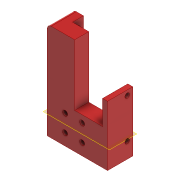
# Autodesk Inventor part: Collector mount adapter
Saved by Autodesk Inventor 2020 (Build 240168000, 168)
## iProperties
Created: 2020-01-01
Part Number: Collector mount adapter
Material: Generic
Document SubType Name: Modeling
Designer: ball
Density: 1 g/cm^3
Appearance: Default
Author: ball
Autodesk Inventor part; units mm, degrees
ref_plane "YZ Plane" through (0, 0, 0) normal (1, 0, 0) x (0, 1, 0)
ref_plane "XZ Plane" through (0, 0, 0) normal (0, 1, 0) x (-1, 0, 0)
ref_plane "Work Plane1" through (0, 0, 0) normal (0, 0, 1) x (1, 0, 0)
sketch "Sketch1" plane through (0, 0, 0) normal (0, 0, 1) x (1, 0, 0)
  line L0 (-13.625, 22.3146) -> (-10.375, 22.3146) construction
  line L1 (3.2502, 80.8) -> (3.2502, 93.5) construction
  line L2 (14.75, 68.1) -> (10.0002, 68.1) construction
  circle A0 centre (12.375, 55.8) radius 3.5 construction
  circle A1 centre (12.375, 47.8) radius 1.7 construction
  line L3 (-18.004, 18.76) -> (18.004, 18.76)
  line L4 (18.004, 18.76) -> (18.004, 47.8)
  line L5 (18.004, 47.8) -> (-4.75, 47.8)
  line L6 (-18.004, 47.8) -> (-18.004, 18.76)
  line L7 (-1.55, 84.1622) -> (-1.55, 90.1378) construction
  line L8 (-4.75, 85.6895) -> (-4.75, 88.6105) construction
  line L9 (17.75, 97.5) -> (-17.75, 97.5) construction
  line L10 (-4.75, 47.8) -> (-4.75, 97.5)
  line L11 (-4.75, 97.5) -> (-18.004, 97.5)
  line L12 (-18.004, 97.5) -> (-18.004, 47.8)
  point P0 (0, 0)
  dimension "d51" = 18.004
  dimension "d52" = 18.004
  dimension "d78" = 97.5
  dimension "d79" = 78.74
  constraints: 26 end point, 4 horizontal, 3 parallel, 3 vertical, 2 centre point, 1 perpendicular, 1 point on line, 16 other
  measures "d51" distance from line of L6 point (0, 0)
  measures "d52" distance from line of L4 point (0, 0)
  measures "d78" distance from line of L9 point (0, 0)
  measures "d79" distance between parallel lines of L3 L9
extrude "Base shape" add sketch "Sketch1" along normal blind 11.4808
sketch "Sketch4" plane through (-18.004, 18.76, 0) normal (-1, 0, 0) x (0, 0, 1)
  line L0 (0, 78.74) -> (11.4808, 78.74) projected
  line L1 (11.4808, 78.74) -> (-8.9916, 78.74)
  line L2 (-8.9916, 78.74) -> (-8.9916, 0)
  line L3 (-8.9916, 0) -> (11.4808, 0)
  line L4 (11.4808, 0) -> (11.4808, 78.74)
  circle A0 centre (-4.4958, 72.0852) radius 1.9
  line L5 (0, 78.74) -> (0, 0) projected
  circle A1 centre (-4.4958, 44.8056) radius 1.9
  circle A2 centre (-4.4958, 12.74) radius 1.9
  point P0 (0, -18.76)
  dimension "d29" = 3.8
  dimension "d30" = 6.6548
  dimension "d32" = 4.4958
  dimension "d33" = 3.8
  dimension "d34" = 3.8
  dimension "d35" = 33.9344
  dimension "d36" = 66
  dimension "d53" = 8.9916
  dimension "d54" = 4.4958
  dimension "d55" = 4.4958
  constraints: 8 end point, 3 centre point, 2 parallel, 1 horizontal, 1 perpendicular
  measures "d29" diameter of A0
  measures "d30" distance from line of L1 A0.centre
  measures "d32" distance from line of L2 A0.centre
  measures "d33" diameter of A1
  measures "d34" diameter of A2
  measures "d35" distance from line of L1 A1.centre
  measures "d36" distance from line of L1 A2.centre
  measures "d53" distance between parallel lines of L2 L5
  measures "d54" distance from line of L2 A1.centre
  measures "d55" distance from line of L2 A2.centre
extrude "Non Pulley Side" add sketch "Sketch4" along normal blind 9
sketch "Sketch5" plane through (18.004, 18.76, 0) normal (1, 0, 0) x (0, 0, -1)
  line L0 (0, 0) -> (-11.4808, 0) projected
  line L1 (0, 78.74) -> (8.9916, 78.74) projected
  line L2 (-11.4808, 0) -> (8.9916, 0)
  line L3 (8.9916, 0) -> (8.9916, 48.815)
  line L4 (8.9916, 78.74) -> (-9.652, 78.74) construction
  line L5 (-11.4808, 48.815) -> (-11.4808, 0)
  circle A0 centre (4.4958, 12.74) radius 1.9
  circle A1 centre (4.4958, 44.815) radius 1.9
  line L6 (8.9916, 78.74) -> (8.9916, 0) projected
  line L7 (8.9916, 48.815) -> (-11.4808, 48.815)
  point P0 (0, -18.76)
  dimension "d40" = 3.8
  dimension "d42" = 66
  dimension "d43" = 3.8
  dimension "d44" = 33.925
  dimension "d45" = 4.4958
  dimension "d46" = 4.4958
  dimension "d49" = 4
  constraints: 10 end point, 2 centre point, 2 parallel, 2 perpendicular, 1 horizontal, 1 point on line
  measures "d40" diameter of A0
  measures "d42" distance from line of L1 A0.centre
  measures "d43" diameter of A1
  measures "d44" distance from line of L1 A1.centre
  measures "d45" distance from line of L3 A0.centre
  measures "d46" distance from line of L3 A1.centre
  measures "d49" distance from line of L7 A1.centre
extrude "Pulley Side" add sketch "Sketch5" along normal blind 4
sketch "Sketch7" plane through (0, 0, 0) normal (0, 0, -1) x (-1, 0, 0)
  circle A0 centre (5.541, 35.04) radius 9.779 construction
  line L0 (27.004, 97.5) -> (27.004, 18.76) construction
  line L1 (5.541, 35.04) -> (12.4558, 28.1252) construction
  line L2 (5.541, 35.04) -> (15.32, 35.04) construction
  line L3 (36.0056, 35.04) -> (-27.0056, 35.04) projected
  point P0 (0, 0)
  point P1 (12.4558, 41.9548)
  point P2 (-1.3738, 41.9548)
  point P3 (-1.3738, 28.1252)
  dimension "d63" = 19.558
  dimension "d64" = 21.463
  dimension "d65" = 45
  dimension "d66" = 0
  dimension "d69" = 360
  constraints: 4 end point, 1 coincident, 1 equal length, 1 horizontal, 8 other
  measures "d64" distance from line of L1.start L0
  measures "d65" angle of L1 L2
  measures "d66" distance from line of L3 L1.start
hole "Turntable mounting holes" at (-12.4558, 41.9548, 0) at (1.3738, 41.9548, 0) at (1.3738, 28.1252, 0) at (-12.4558, 28.1252, 0) direction (0, 0, 1) diameter 4.064 end through all counterbore diameter 8.89 counterbore depth 5.8928
ref_plane "Work Plane5" through (-12.4558, 35.04, 5.8928) normal (0, 1, 0) x (0, 0, -1)
ref_plane "Work Plane3" through (-12.4558, 28.1252, 5.8928) normal (0, 1, 0) x (0, 0, -1)
ref_plane "Work Plane4" through (-12.4558, 41.9548, 5.8928) normal (0, 1, 0) x (0, 0, -1)
sketch "Sketch6" plane through (-18.004, 18.76, 0) normal (1, 0, 0) x (0, 0, -1)
  line L0 (8.9916, 0) -> (-11.4808, 0) projected
  line L1 (8.9916, 78.74) -> (8.9916, 0) projected
  line L2 (-15.5753, 16.28) -> (13.0861, 16.28) projected
  point P0 (0, -18.76)
  point P1 (4.4958, 6.501)
  point P2 (4.4958, 26.059)
  dimension "d85" = 9.779
  dimension "d86" = 9.779
  dimension "d87" = 4.4958
  dimension "d88" = 4.4958
  measures "d85" distance from line of point (4.496, 6.501) L2
  measures "d86" distance from line of point (4.496, 26.059) L2
  measures "d87" distance from line of point (4.496, 26.059) L1
  measures "d88" distance from line of L1 point (4.496, 6.501)
hole "Servo mounting holes" at (-18.004, 25.261, -4.4958) at (-18.004, 44.819, -4.4958) direction (-1, 0, 0) diameter 4.064 end through all counterbore diameter 8.89 counterbore depth 4.064
fillet "Fillet2" radius 3.175 1 edges at (-27.004, 97.5, 1.2446)
equation "\"d32\" = 0.5 * d31"
equation "\"d33\" = d29"
equation "\"d34\" = d29"
equation "\"d54\" = d32"
equation "\"d55\" = d32"
equation "\"d40\" = d29"
equation "\"d43\" = d29"
equation "\"d45\" = d32"
equation "\"d46\" = d32"
equation "\"d86\" = d85"
equation "\"d88\" = d87"
equation "\"d31\" = 8.9916"
body "Solid1"
